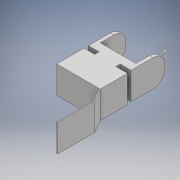
# Autodesk Inventor part: CRANEJ4
Saved by Autodesk Inventor 2017 (Build 210142000, 142)
## iProperties
Part Number: CRANEJ4
Material: 一般
Document SubType Name: Modeling
Designer: rsdlab
Density: 1 g/cm^3
Appearance: 既定
Author: rsdlab
Autodesk Inventor part; units mm, degrees
ref_plane "YZ Plane" through (0, 0, 0) normal (1, 0, 0) x (0, 1, 0)
ref_plane "XZ Plane" through (0, 0, 0) normal (0, 1, 0) x (-1, 0, 0)
ref_plane "XY Plane" through (0, 0, 0) normal (0, 0, 1) x (1, 0, 0)
sketch "スケッチ1" plane through (0, 0, 0) normal (0, 1, 0) x (-1, 0, 0)
  line L0 (0, 0) -> (0.04, 0)
  line L1 (0.04, 0) -> (0.04, -0.32)
  line L2 (0.04, -0.32) -> (0, -0.32)
  line L3 (0, -0.32) -> (0, 0)
  line L4 (0.46, 0) -> (0.5, 0)
  line L5 (0.5, 0) -> (0.5, -0.32)
  line L6 (0.5, -0.32) -> (0.46, -0.32)
  line L7 (0.46, -0.32) -> (0.46, 0)
  dimension "d0" = 0.04
  dimension "d1" = 0.32
  dimension "d2" = 0.04
  constraints: 16 end point, 4 parallel, 2 horizontal, 2 perpendicular
  measures "d0" distance of L1.end L2.end
  measures "d1" distance of L0.end L1.end
  measures "d2" distance of L5.end L6.end
extrude "押し出し1" add sketch "スケッチ1" against normal blind 0.3
sketch "スケッチ2" plane through (0, -0.3, 0) normal (0, -1, 0) x (1, 0, 0)
  line L0 (0, -0.32) -> (0, 0) projected
  line L1 (-0.5, 0) -> (-0.5, -0.32) projected
  line L2 (0, 0) -> (-0.5, 0)
  line L3 (-0.5, 0) -> (-0.5, -0.32)
  line L4 (-0.5, -0.32) -> (0, -0.32)
  line L5 (0, -0.32) -> (0, 0)
  constraints: 8 end point, 2 parallel, 1 horizontal, 1 perpendicular
extrude "押し出し2" add sketch "スケッチ2" along normal blind 0.1
sketch "スケッチ3" plane through (0, -0.4, 0) normal (0, -1, 0) x (1, 0, 0)
  line L0 (-0.04, 0) -> (-0.46, 0) projected
  line L1 (-0.46, -0.32) -> (-0.04, -0.32) projected
  line L2 (-0.125, 0) -> (-0.375, 0)
  line L3 (-0.375, 0) -> (-0.375, -0.32)
  line L4 (-0.375, -0.32) -> (-0.125, -0.32)
  line L5 (-0.125, -0.32) -> (-0.125, 0)
  point P0 (0, 0)
  dimension "d7" = 0.25
  constraints: 8 end point, 2 parallel, 2 point on line, 1 horizontal, 1 perpendicular
  measures "d7" distance of L4.end L3.end
extrude "押し出し3" add sketch "スケッチ3" along normal blind 0.05
sketch "スケッチ4" plane through (0, -0.45, 0) normal (0, -1, 0) x (1, 0, 0)
  line L0 (-0.5, 0) -> (-0.5, -0.32) projected
  line L1 (0, 0) -> (-0.5, 0)
  line L2 (-0.5, 0) -> (-0.5, -0.32)
  line L3 (-0.5, -0.32) -> (0, -0.32)
  line L4 (0, -0.32) -> (0, 0)
  constraints: 8 end point, 2 parallel, 1 horizontal, 1 perpendicular
extrude "押し出し4" add sketch "スケッチ4" along normal blind 0.32
sketch "スケッチ5" plane through (0, -0.45, 0) normal (1, 0, 0) x (0, 0, -1)
  line L0 (0.32, 0) -> (0.32, -0.32) projected
  line L1 (0, 0) -> (0.32, 0)
  line L2 (0.32, 0) -> (0.32, -0.32)
  line L3 (0.32, -0.32) -> (0, -0.32)
  line L4 (0, -0.32) -> (0, 0)
  point P0 (0, 0.45)
  constraints: 8 end point, 2 parallel, 1 horizontal, 1 perpendicular
extrude "押し出し5" add sketch "スケッチ5" along normal blind 0.01
sketch "スケッチ6" plane through (0, -0.77, 0) normal (0, -1, 0) x (1, 0, 0)
  line L0 (0, -0.32) -> (0, 0) projected
  line L1 (0, 0) -> (0.1, 0)
  line L2 (0.1, 0) -> (0.1, -0.32)
  line L3 (0.1, -0.32) -> (0, -0.32)
  line L4 (0, -0.32) -> (0, 0)
  dimension "d14" = 0.1
  constraints: 8 end point, 2 parallel, 1 horizontal, 1 perpendicular
  measures "d14" distance of L2.end L3.end
extrude "押し出し6" add sketch "スケッチ6" along normal blind 0.16
chamfer "面取り1" distance 0.09 distance2 0.16 1 edges at (0, -0.93, -0.16) measured on face at (0.0333, -0.93, -0.1067)
chamfer "面取り2" distance 0.09 distance2 0.16 1 edges at (0.1, -0.77, -0.16) measured on face at (0.04, -0.77, -0.1067)
sketch "スケッチ7" plane through (0, -0.93, 0) normal (0, -1, 0) x (1, 0, 0)
  line L0 (0.1, -0.32) -> (0.1, 0) projected
  line L1 (0, -0.32) -> (0.09, -0.32) projected
  line L2 (0.1, 0) -> (0.09, 0)
  line L3 (0.09, 0) -> (0.09, -0.32)
  line L4 (0.09, -0.32) -> (0.1, -0.32)
  line L5 (0.1, -0.32) -> (0.1, 0)
  point P0 (0, 0)
  constraints: 8 end point, 2 parallel, 1 horizontal, 1 perpendicular
extrude "押し出し7" add sketch "スケッチ7" along normal blind 0.43
fillet "フィレット1" radius 0.14 4 edges at (-0.02, 0, 0) (-0.02, 0, -0.32) (-0.48, 0, 0) (-0.48, 0, -0.32)
sketch "スケッチ8" plane through (-0.46, -0.3, 0) normal (0, 0, 1) x (1, 0, 0)
  point P0 (0.46, 0.3)
